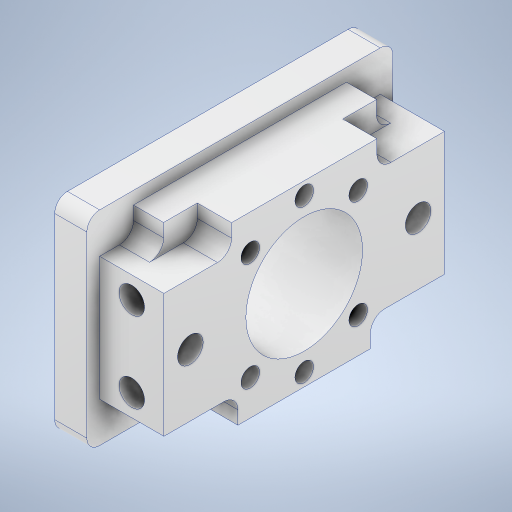
# Autodesk Inventor part: BS_Face
Saved by Autodesk Inventor 2023 (Build 270158000, 158)
## iProperties
Created: 2025-04-19
Part Number: BS_Face
Material: Aluminum 6061
Document SubType Name: Modeling
Designer: plebbb
Density: 2.7 g/cm^3
Appearance: Aluminum - Flat
Author: plebbb
Autodesk Inventor part; units mm, degrees
ref_plane "YZ Plane" through (0, 0, 0) normal (1, 0, 0) x (0, 1, 0)
ref_plane "XZ Plane" through (0, 0, 0) normal (0, 1, 0) x (-1, 0, 0)
sketch "Sketch1" plane through (0, 0, 0) normal (1, 0, 0) x (0, 1, 0)
  line L0 (0, 0) -> (50.8, 0) construction
  line L1 (50.8, 0) -> (50.8, 76.2) construction
  line L2 (50.8, 76.2) -> (0, 76.2) construction
  line L3 (0, 76.2) -> (0, 0) construction
  line L4 (40.8, 3.175) -> (10, 3.175)
  line L5 (10, 3.175) -> (10, 11.6)
  line L6 (10, 11.6) -> (3.175, 11.6)
  line L7 (3.175, 11.6) -> (3.175, 64.6)
  line L8 (3.175, 64.6) -> (10, 64.6)
  line L9 (10, 64.6) -> (10, 73.025)
  line L10 (10, 73.025) -> (40.8, 73.025)
  line L11 (40.8, 73.025) -> (40.8, 64.6)
  line L12 (40.8, 64.6) -> (47.625, 64.6)
  line L13 (47.625, 64.6) -> (47.625, 11.6)
  line L14 (47.625, 11.6) -> (40.8, 11.6)
  line L15 (40.8, 3.175) -> (40.8, 11.6)
  line L16 (25.4, 73.025) -> (25.4, 76.2) construction
  line L17 (47.625, 38.1) -> (50.8, 38.1) construction
  line L18 (3.175, 38.1) -> (0, 38.1) construction
  line L19 (25.4, 3.175) -> (25.4, 0) construction
  point P0 (1.5875, 38.1)
  dimension "d0" = 50.8
  dimension "d1" = 76.2
  dimension "d2" = 3.175
  dimension "d3" = 26.5
  dimension "d4" = 10
  constraints: 40 end point, 10 perpendicular, 9 midpoint, 6 equal length, 5 point on line, 3 parallel, 2 horizontal
  measures "d0" distance of L0.start L0.end
  measures "d1" distance of L0.end L1.end
  measures "d2" distance of L16.start L16.end
  measures "d3" distance from line of point (1.587, 38.1) L8
  measures "d4" horizontal distance of L2.end L8.end
extrude "Extrusion1" add sketch "Sketch1" along normal blind 16
sketch "Sketch2" plane through (0, 10, 73.025) normal (0, 0, 1) x (1, 0, 0)
  line L0 (0, -10) -> (16, -10) construction
  line L1 (16, -10) -> (16, 40.8) construction
  line L2 (16, 40.8) -> (0, 40.8) construction
  line L3 (0, 40.8) -> (0, -10) construction
  circle A0 centre (8, 25.4) radius 3.175
  circle A1 centre (8, 5.4) radius 3.175
  line L4 (8, 25.4) -> (8, 40.8) construction
  line L5 (8, 5.4) -> (8, -10) construction
  dimension "d7" = 16
  dimension "d8" = 50.8
  dimension "d9" = 6.35
  dimension "d10" = 20
  constraints: 12 end point, 3 perpendicular, 2 centre point, 2 midpoint, 2 parallel, 1 collinear, 1 equal radius, 1 horizontal
  measures "d7" distance of L1.end L2.end
  measures "d8" distance of L0.end L1.end
  measures "d9" diameter of A0
  measures "d10" distance of L5.start L4.start
extrude "Extrusion2" cut sketch "Sketch2" against normal blind 16
ref_plane "Work Plane1" through (0, 10, 38.1) normal (0, 0, 1) x (1, 0, 0)
mirror "Mirror1" about plane through (0, 10, 38.1) normal (0, 0, 1) of "Extrusion2"
sketch "Sketch5" plane through (0, 47.625, 64.6) normal (0, 1, 0) x (1, 0, 0)
  line L0 (0, 64.6) -> (16, 64.6) construction
  line L1 (16, 64.6) -> (16, -11.6) construction
  line L2 (16, -11.6) -> (0, -11.6) construction
  line L3 (0, -11.6) -> (0, 64.6) construction
  line L4 (12.5, 3.4) -> (12.5, -11.6) construction
  line L5 (12.5, 49.6) -> (12.5, 64.6) construction
  line L6 (7.5, 8.4) -> (16, 8.4)
  line L7 (16, 8.4) -> (16, -11.6)
  line L8 (16, -11.6) -> (7.5, -11.6)
  line L9 (7.5, -11.6) -> (7.5, 8.4)
  line L10 (12.5, 3.4) -> (7.5, 3.4) construction
  line L11 (12.5, 3.4) -> (16, 3.4) construction
  line L12 (12.5, 3.4) -> (12.5, 8.4) construction
  line L13 (7.5, 44.6) -> (16, 44.6)
  line L14 (16, 44.6) -> (16, 64.6)
  line L15 (16, 64.6) -> (7.5, 64.6)
  line L16 (7.5, 64.6) -> (7.5, 44.6)
  line L17 (12.5, 49.6) -> (12.5, 44.6) construction
  line L18 (12.5, 49.6) -> (7.5, 49.6) construction
  dimension "d18" = 76.2
  dimension "d19" = 16
  dimension "d21" = 15
  dimension "d22" = 12.5
  dimension "d23" = 5
  constraints: 38 end point, 10 perpendicular, 8 point on line, 6 parallel, 4 equal length, 3 horizontal
  measures "d18" distance of L2.end L0.start
  measures "d19" distance of L0.start L0.end
  measures "d21" distance of L4.start L4.end
  measures "d22" distance from line of L3 L4.start
  measures "d23" distance of L4.start L10.end
extrude "Extrusion4" cut sketch "Sketch5" against normal up to surface (6.825 mm away)
sketch "Sketch6" plane through (0, 3.175, 11.6) normal (0, -1, 0) x (1, 0, 0)
  line L0 (0, -11.6) -> (16, -11.6) construction
  line L1 (16, -11.6) -> (16, 64.6) construction
  line L2 (16, 64.6) -> (0, 64.6) construction
  line L3 (0, 64.6) -> (0, -11.6) construction
  line L4 (10, 53) -> (10, 0) construction
  line L5 (10, 26.5) -> (0, 26.5) construction
  line L6 (16, 43) -> (0, 43)
  line L7 (0, 43) -> (0, 64.6)
  line L8 (0, 64.6) -> (16, 64.6)
  line L9 (16, 64.6) -> (16, 43)
  line L10 (16, 10) -> (0, 10)
  line L11 (0, 10) -> (0, -11.6)
  line L12 (0, -11.6) -> (16, -11.6)
  line L13 (16, -11.6) -> (16, 10)
  dimension "d26" = 16
  dimension "d27" = 76.2
  dimension "d28" = 10
  dimension "d29" = 53
  dimension "d30" = 10
  constraints: 28 end point, 6 parallel, 4 perpendicular, 3 horizontal, 2 midpoint, 2 point on line, 1 collinear, 1 vertical
  measures "d26" distance of L0.start L0.end
  measures "d27" distance of L0.end L1.end
  measures "d28" distance of L5.start L5.end
  measures "d29" distance of L4.start L4.end
  measures "d30" distance from line of L6 L4.start
extrude "Extrusion5" cut sketch "Sketch6" against normal up to surface (6.825 mm away)
fillet "Fillet1" radius 3.5 6 edges at (8, 10, 54.6) (3.75, 40.8, 64.6) (11.75, 40.8, 56.2) (3.75, 40.8, 11.6) (11.75, 40.8, 20) (8, 10, 21.6)
sketch "Sketch4" plane through (0, 0, 0) normal (-1, 0, 0) x (0, 0, 1)
  line L0 (0, 0) -> (76.2, 0)
  line L1 (76.2, 0) -> (76.2, 50.8)
  line L2 (76.2, 50.8) -> (0, 50.8)
  line L3 (0, 50.8) -> (0, 0)
  dimension "d13" = 76.2
  dimension "d14" = 50.8
  constraints: 8 end point, 2 parallel, 1 horizontal, 1 perpendicular
  measures "d13" distance of L1.end L2.end
  measures "d14" distance of L0.end L1.end
extrude "Extrusion3" add sketch "Sketch4" along normal blind 8
sketch "Sketch7" plane through (-8, 0, 0) normal (-1, 0, 0) x (0, 0, 1)
  circle A0 centre (38.1, 25.4) radius 14.5
  circle A1 centre (38.1, 25.4) radius 19 construction
  circle A2 centre (24.665, 38.835) radius 2.3
  circle A3 centre (38.1, 44.4) radius 2.3
  circle A4 centre (24.665, 11.965) radius 2.3
  circle A5 centre (38.1, 6.4) radius 2.3
  circle A6 centre (51.535, 38.835) radius 2.3
  circle A7 centre (51.535, 11.965) radius 2.3
  line L0 (51.535, 38.835) -> (38.1, 25.4) construction
  line L1 (38.1, 25.4) -> (38.1, 44.4) construction
  line L2 (0, 0) -> (76.2, 0) construction
  line L3 (76.2, 0) -> (76.2, 50.8) construction
  line L4 (76.2, 50.8) -> (0, 50.8) construction
  line L5 (0, 50.8) -> (0, 0) construction
  circle A8 centre (9.75, 25.4) radius 3.175
  circle A9 centre (66.45, 25.4) radius 3.175
  line L6 (9.75, 25.4) -> (0, 25.4) construction
  line L7 (66.45, 25.4) -> (76.2, 25.4) construction
  circle A10 centre (38.1, 25.4) radius 25 construction
  line L8 (18.1, 25.4) -> (9.75, 25.4) construction
  line L9 (38.1, 25.4) -> (18.1, 25.4) construction
  point P0 (38.1, 50.8)
  dimension "d37" = 29
  dimension "d38" = 38
  dimension "d39" = 4.6
  dimension "d40" = 45
  dimension "d41" = 76.2
  dimension "d42" = 50.8
  dimension "d43" = 6.35
  dimension "d44" = 6.35
  dimension "d45" = 50
  dimension "d51" = 20
  dimension "d52" = 8.35
  constraints: 20 end point, 11 centre point, 6 point on circle, 5 equal radius, 3 coincident, 3 horizontal, 3 midpoint, 3 perpendicular, 3 vertical alignment, 2 horizontal alignment, 2 parallel, 1 collinear, 1 point on line, 1 vertical
  measures "d37" diameter of A0
  measures "d38" diameter of A1
  measures "d39" diameter of A3
  measures "d40" angle of L1 L0
  measures "d41" distance of L3.end L4.end
  measures "d42" distance of L2.end L3.end
  measures "d43" diameter of A8
  measures "d44" diameter of A9
  measures "d45" diameter of A10
  measures "d51" distance of L0.end L8.start
  measures "d52" distance of L8.start L6.start
extrude "Extrusion6" cut sketch "Sketch7" against normal through all
fillet "Fillet2" radius 3.175 4 edges at (-4, 50.8, 0) (-4, 50.8, 76.2) (-4, 0, 76.2) (-4, 0, 0)
body "Solid1"
